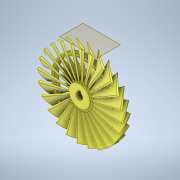
# Autodesk Inventor part: newRotor.24.1.0
Saved by Autodesk Inventor 2021.2 (Build 252289000, 289)
## iProperties
Created: 2021-05-16
Part Number: newRotor.24.1.0
Material: Generic
Document SubType Name: Modeling
Designer: Ryan
Density: 1 g/cm^3
Appearance: Smooth - Yellow
Author: Ryan
## iProperties of the stored document _3DPrint.ipt
Created: 2021-05-23
Part Number: _3DPrint
Material: Generic
Document SubType Name: Modeling
Designer: Ryan
Density: 1 g/cm^3
Appearance: Default
Author: Ryan
Autodesk Inventor part; units mm, degrees
ref_plane "YZ Plane" through (0, 0, 0) normal (1, 0, 0) x (0, 1, 0)
ref_plane "XY Plane" through (0, 0, 0) normal (0, 0, 1) x (1, 0, 0)
sketch "Sketch1" plane through (0, 0, 0) normal (0, 0, 1) x (1, 0, 0)
  circle A0 centre (0, 0) radius 12.7
  dimension "d0" = 25.4
  constraints: 1 centre point, 1 coincident
  measures "d0" diameter of A0
extrude "Extrusion1" add sketch "Sketch1" against normal blind 25.4 draft 11.31
ref_plane "Work Plane1" through (0, 15.24, 0) normal (0, 1, 0) x (-1, 0, 0)
ref_plane "Work Plane2" through (0, 50.8, 0) normal (0, 1, 0) x (-1, 0, 0)
sketch "Sketch5" plane through (0, 15.24, 0) normal (0, 1, 0) x (-1, 0, 0)
  line L0 (12.7, 0) -> (17.78, -25.4) projected
  line L1 (15.24, -12.7) -> (18.348, -12.7)
  line L2 (12.7, 0) -> (-12.7, 0) projected
  line L3 (0, 0) -> (0, -26.8939)
  arc A0 (-2.0796, -0.0899) -> (-2.7066, -1.2672) centre (-2.4141, -0.6673) ccw
  arc A1 (1.8548, -11.9063) -> (-2.0796, -0.0899) centre (-11.2756, -9.7149) ccw
  arc A2 (1.8548, -11.9063) -> (-2.7066, -1.2672) centre (-12.357, -11.702) ccw
  line L4 (15.24, -12.7) -> (-15.24, -12.7)
  line L5 (-12.7, 0) -> (-17.78, -25.4) projected
  line L6 (8.4358, -11.1125) -> (0, -11.1125)
  point P0 (1.844, -11.1125)
  point P1 (1.9628, -11.1125)
  point P2 (0, -2.639)
  point P3 (0, -4.6791)
  dimension "d75" = 0.7937
  dimension "d76" = 1.5875
  dimension "d98" = 4.2688
  dimension "d99" = 0.6673
  dimension "d100" = 13.312
  dimension "d101" = 14.2132
  dimension "d102" = 11.2389
  dimension "d103" = 1.1773
  dimension "d104" = 0.627
  constraints: 8 end point, 6 point on circle, 3 centre point, 2 horizontal, 2 midpoint, 1 point on line, 1 vertical
  measures "d75" distance from line of L4 A1.start
  measures "d76" distance between parallel lines of L4 L6
  measures "d98" horizontal distance of A0.centre A1.start
  measures "d99" radius of A0
  measures "d100" radius of A1
  measures "d101" radius of A2
  measures "d102" vertical distance of A0.centre A1.start
  measures "d103" vertical distance of A1.end A0.end
  measures "d104" horizontal distance of A0.end A1.end
sketch "Sketch6" plane through (0, 50.8, 0) normal (0, 1, 0) x (-1, 0, 0)
  line L0 (12.7, 0) -> (-12.7, 0) projected
  line L1 (-12.7, 0) -> (-17.78, -25.4) projected
  line L2 (17.78, -25.4) -> (-17.78, -25.4) projected
  line L3 (0, -25.4) -> (0, 15.7367)
  arc A0 (-2.4165, -0.3662) -> (-3.6441, -2.4123) centre (-3.0351, -1.3864) ccw
  line L4 (-12.7, 0) -> (-17.78, -25.4) projected
  line L5 (-15.24, -12.7) -> (33.5524, -12.7)
  arc A1 (14.9286, -11.1125) -> (-3.6441, -2.4123) centre (-24.5745, -71.2672) ccw
  line L6 (15.2055, -11.1125) -> (14.9286, -11.1125)
  arc A2 (15.2055, -11.1125) -> (-2.4165, -0.3662) centre (-23.0759, -54.0657) ccw
  point P0 (0, 0)
  dimension "d82" = 1.5875
  dimension "d106" = 71.9658
  dimension "d107" = 1.1931
  dimension "d108" = 17.9637
  dimension "d109" = 18.2406
  dimension "d112" = 1.3864
  dimension "d113" = 0.2769
  dimension "d114" = 57.5365
  dimension "d115" = 2.0461
  dimension "d116" = 1.2276
  constraints: 7 point on circle, 6 end point, 3 centre point, 2 horizontal, 2 midpoint, 1 vertical
  measures "d82" distance between parallel lines of L6 L5
  measures "d106" radius of A1
  measures "d107" radius of A0
  measures "d108" horizontal distance of A1.start A0.centre
  measures "d109" horizontal distance of A0.centre L6.start
  measures "d112" distance from line of L0 A0.centre
  measures "d113" distance of L6.start L6.end
  measures "d114" radius of A2
  measures "d115" vertical distance of A0.start A0.end
  measures "d116" horizontal distance of A0.end A0.start
sketch "Sketch8" plane through (0, 0, 0) normal (0, 0, 1) x (1, 0, 0)
  circle A0 centre (0, 0) radius 4
  line L0 (-1.5875, 5.5875) -> (1.5875, 5.5875)
  line L1 (1.5875, 5.5875) -> (1.5875, 2.4125)
  line L2 (1.5875, 2.4125) -> (-1.5875, 2.4125)
  line L3 (-1.5875, 2.4125) -> (-1.5875, 5.5875)
  line L4 (-1.5875, 5.5875) -> (1.5875, 2.4125) construction
  line L5 (1.5875, 5.5875) -> (-1.5875, 2.4125) construction
  point P0 (0, 4)
  point P1 (-1.5875, 3.6715)
  point P2 (1.5875, 3.6715)
  dimension "d39" = 8
  dimension "d40" = 3.175
  dimension "d41" = 3.175
  constraints: 12 end point, 2 midpoint, 2 parallel, 1 coincident, 1 horizontal, 1 perpendicular, 3 other
  measures "d40" distance of L1.end L2.end
  measures "d41" distance of L0.end L1.end
extrude "Extrusion5" cut sketch "Sketch8" against normal through all
sketch "Sketch13" plane through (0, 0, 0) normal (0, 0, 1) x (1, 0, 0)
  circle A0 centre (0, 0) radius 12.7 projected
  circle A1 centre (0, 0) radius 50.0063
  arc A2 (-1.5875, 3.6715) -> (1.5875, 3.6715) centre (0, 0) ccw projected
  circle A3 centre (0, 0) radius 80.6636
  dimension "d66" = 100.0125
  constraints: 2 centre point, 2 coincident
  measures "d66" diameter of A1
extrude "Extrusion7" add sketch "Sketch5" against normal blind 5.08 contours A0 A1 L3 A2 | A1 L6 A2 L3
loft "Loft5" add profiles "Sketch6" section 1 edges at (-1.2224, 15.24, -5.1315) (3.0031, 15.24, -0.3536) (-0.5447, 15.24, -5.7387) (-1.9034, 15.24, -11.1125) contours A2 L6 A1 L3 | L3 A1 A0 A2
sketch "Sketch14" plane through (0, 0, 0) normal (1, 0, 0) x (0, 1, 0)
  line L0 (36.83, -3.7163) -> (36.1962, -3.7163)
  line L1 (34.9262, -4.9863) -> (34.9262, -10.1175)
  line L2 (36.2307, -11.3871) -> (36.8645, -11.3698)
  line L3 (38.1, -10.1003) -> (38.1, -4.9863)
  line L4 (50.8, 2.2751) -> (50.8, -13.6506) projected
  arc A0 (38.1, -4.9863) -> (36.83, -3.7163) centre (36.83, -4.9863) ccw
  arc A1 (36.8645, -11.3698) -> (38.1, -10.1003) centre (36.83, -10.1003) ccw
  arc A2 (34.9262, -10.1175) -> (36.2307, -11.3871) centre (36.1962, -10.1175) ccw
  arc A3 (36.1962, -3.7163) -> (34.9262, -4.9863) centre (36.1962, -4.9863) ccw
  line L5 (17.1324, -11.9063) -> (46.331, -11.1125) projected
  line L6 (0, -13.6506) -> (0, 2.2751) projected
  point P0 (0, 0)
  point P1 (38.1, -3.7163)
  point P2 (34.9262, -11.4225)
  point P3 (38.1, -11.3363)
  point P4 (12.7237, -11.1125)
  point P5 (41.9316, -11.1125)
  dimension "d90" = 7.62
  dimension "d91" = 3.175
  dimension "d92" = 12.7
  dimension "d93" = 1.27
  dimension "d94" = 0
  constraints: 8 end point, 8 point on circle, 8 tangent, 6 point on line, 4 centre point, 3 equal radius, 1 horizontal, 1 parallel, 1 perpendicular, 2 other
  measures "d90" distance of point (38.1, -11.336) point (38.1, -3.716)
  measures "d91" distance of point (34.926, -11.423) point (38.1, -11.336)
  measures "d92" distance between parallel lines of L3 L4
  measures "d93" radius of A0
revolve "Revolution5" add sketch "Sketch14" angle 360 about axis through (0, 0, -10) along (0, 0, 1)
pattern_circular "Circular Pattern7" count 24 over 360 about axis through (0, 0, 0) along (0, 0, -1) of "Loft5", "Extrusion7"
extrude "Extrusion9" cut sketch "Sketch13" against normal through all contours A3
body "Solid1"
